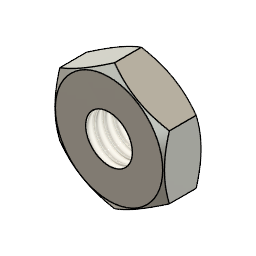
dual_stroke_vacuum_generator (Autodesk Fusion 360 archive; units mm, degrees)
design "Chamfered Bottom Hex Machine Screw Nut ANSI B18.6.3 - 10-32 Steel Grade 2H Plain"
description: Chamfered Bottom Hex Machine Screw Nut ANSI B18.6.3 - 10-32
part number: CBHMSN ANSI B18.6.3 - 10-32 Steel Grade 2H Plain
Autodesk Fusion 360 part; units mm, degrees
note: some values were not read from the file. Chosen so that the rebuilt part matches the saved one: how an offset face is resized.
sketch "Sketch1" plane through (0, 0, 0) normal (0, 1, 0) x (1, 0, 0)
  line L0 (0, 0) -> (0, -3.302)
  line L1 (-2.413, 0) -> (-4.6673, 0)
  line L2 (-4.6673, 0) -> (-5.4991, -0.4803)
  line L3 (-5.4991, -0.4803) -> (-5.4991, -2.8217)
  line L4 (-5.4991, -2.8217) -> (-4.6673, -3.302)
  line L5 (-4.6673, -3.302) -> (-2.413, -3.302)
  line L6 (-2.413, -3.302) -> (-2.413, 0)
  dimension "d121" = 4.826
  dimension "d122" = 30
  dimension "d123" = 30
  dimension "d128" = 10.9982
  dimension "d142" = 9.3345
  dimension "d146" = 3.302
  constraint vertical L0
  constraint coincident L0 L0.end
  constraint coincident origin L0
  constraint horizontal L1
  constraint coincident L0.start L1
  constraint coincident L0.start origin
  constraint vertical L1.end L4.end
  constraint coincident L0.end L5
  measures "d122" angle of L1 L2
  measures "d123" angle of L4 L5
  measures "d146" distance of L1 L5
revolve "Revolve1" add sketch "Sketch1" angle 360 about axis through (0, 0, 0) along (0, 0, 1)
sketch "Sketch8" plane through (0, 0, 3.302) normal (0, 0, 1) x (1, 0, 0)
  line L0 (-4.7625, -2.7493) -> (-4.7625, 2.7493)
  circle A0 centre (0, 0) radius 2.413
  circle A1 centre (0, 0) radius 5.4991
  dimension "d114" = 4.7625
  constraint coincident L0.end A1
  constraint coincident L0.start A1
  constraint vertical L0
  measures "d114" distance of A0.centre L0
extrude "Extrude5" cut sketch "Sketch8" against normal blind 3.302 contours L0 A1 picked at (-4.8813, 0.6696)
pattern_circular "C-Pattern2" count 6 over 360 about axis through (0, 0, 1.75) along (0, 0, 1) of "Extrude5"
thread "Thread3" "ANSI Unified Screw Threads 0.19(#10) 10-32 UNF 10-32 UNF 2B" major diameter 4.826 minor diameter 4.064 pitch 0.7937 angle 60 resizes the face on face at (-2.41, 0.1203, 2.2013)
equation "d89 = -adsk_nheig"
equation "d114 = adsk_waflat / 2"
equation "adsk_chamang1 = 30 deg"
equation "adsk_chamang2 = 30 deg"
equation "d121 = adsk_nomdia"
equation "d122 = adsk_chamang1"
equation "d123 = adsk_chamang2"
equation "d128 = adsk_maxdia"
equation "adsk_nheig = 0.13 in"
equation "adsk_maxdia = 0.433 in"
equation "adsk_nomdia = 0.19 in"
equation "adsk_waflat = 0.375 in"
equation "d139 = adsk_nheig"
equation "adsk_beardia = adsk_waflat * 0.98"
equation "d142 = adsk_beardia"
equation "d146 = adsk_nheig"

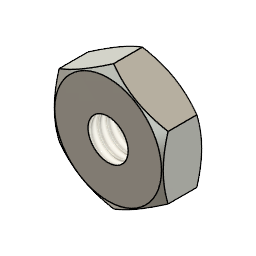
design "Chamfered Bottom Hex Machine Screw Nut ANSI B18.6.3 - 6-40 Steel Grade 2H Plain"
description: Chamfered Bottom Hex Machine Screw Nut ANSI B18.6.3 - 6-40
part number: CBHMSN ANSI B18.6.3 - 6-40 Steel Grade 2H Plain
Autodesk Fusion 360 part; units mm, degrees
sketch "Sketch1" plane through (0, 0, 0) normal (0, 1, 0) x (1, 0, 0)
  line L0 (0, 0) -> (0, -2.8956)
  line L1 (-1.7526, 0) -> (-3.8832, 0)
  line L2 (-3.8832, 0) -> (-4.5847, -0.405)
  line L3 (-4.5847, -0.405) -> (-4.5847, -2.4906)
  line L4 (-4.5847, -2.4906) -> (-3.8832, -2.8956)
  line L5 (-3.8832, -2.8956) -> (-1.7526, -2.8956)
  line L6 (-1.7526, -2.8956) -> (-1.7526, 0)
  dimension "d121" = 3.5052
  dimension "d122" = 30
  dimension "d123" = 30
  dimension "d128" = 9.1694
  dimension "d142" = 7.7663
  dimension "d146" = 2.8956
  constraint vertical L0
  constraint coincident L0 L0.end
  constraint coincident origin L0
  constraint horizontal L1
  constraint coincident L0.start L1
  constraint coincident L0.start origin
  constraint vertical L1.end L4.end
  constraint coincident L0.end L5
  measures "d122" angle of L1 L2
  measures "d123" angle of L4 L5
  measures "d146" distance of L1 L5
revolve "Revolve1" add sketch "Sketch1" angle 360 about axis through (0, 0, 0) along (0, 0, 1)
sketch "Sketch8" plane through (0, 0, 2.8956) normal (0, 0, 1) x (1, 0, 0)
  line L0 (-3.9624, -2.3063) -> (-3.9624, 2.3063)
  circle A0 centre (0, 0) radius 1.7526
  circle A1 centre (0, 0) radius 4.5847
  dimension "d114" = 3.9624
  constraint coincident L0.end A1
  constraint coincident L0.start A1
  constraint vertical L0
  measures "d114" distance of A0.centre L0
extrude "Extrude5" cut sketch "Sketch8" against normal blind 2.8956 contours L0 A1 picked at (-4.052, -0.5885)
pattern_circular "C-Pattern2" count 6 over 360 about axis through (0, 0, 1.75) along (0, 0, 1) of "Extrude5"
thread "Thread3" "ANSI Unified Screw Threads 0.138(#6) 6-40 UNF 6-40 UNF 2B" major diameter 3.5052 minor diameter 2.921 pitch 0.635 angle 60 resizes the face on face at (-1.7439, 0.1745, 0.9652)
equation "d89 = -adsk_nheig"
equation "d114 = adsk_waflat / 2"
equation "adsk_chamang1 = 30 deg"
equation "adsk_chamang2 = 30 deg"
equation "d121 = adsk_nomdia"
equation "d122 = adsk_chamang1"
equation "d123 = adsk_chamang2"
equation "d128 = adsk_maxdia"
equation "adsk_nheig = 0.114 in"
equation "adsk_maxdia = 0.361 in"
equation "adsk_nomdia = 0.138 in"
equation "adsk_waflat = 0.312 in"
equation "d139 = adsk_nheig"
equation "adsk_beardia = adsk_waflat * 0.98"
equation "d142 = adsk_beardia"
equation "d146 = adsk_nheig"
